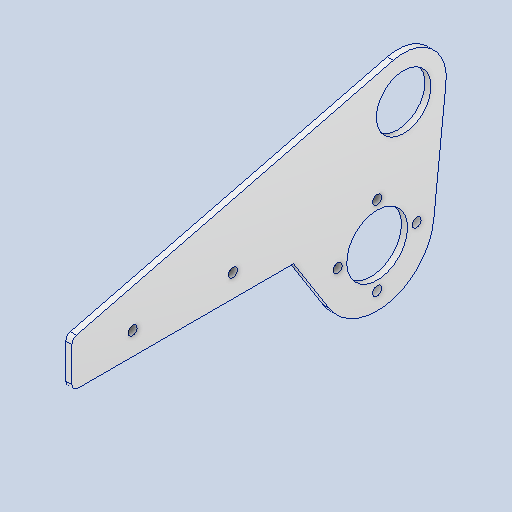
# Autodesk Inventor part: RZvector-arm-rotate-v1-Plate-MM5-F
Saved by Autodesk Inventor 2024 (Build 280153000, 153)
## iProperties
Created: 2024-03-10
Part Number: RZvector-arm-rotate-v1-Plate-MM5-F
Material: アルミニウム 6061
Document SubType Name: Modeling
Designer: haruy
Density: 2.7 g/cm^3
Appearance: アルミニウム - フラット
Mass: 7.93605 g
Surface Area: 89.4411 cm^2
Volume: 7.93605 cm^3
Author: haruy
Autodesk Inventor part; units mm, degrees
ref_plane "YZ Plane" through (0, 0, 0) normal (1, 0, 0) x (0, 1, 0)
ref_plane "XZ Plane" through (0, 0, 0) normal (0, 1, 0) x (-1, 0, 0)
ref_plane "XY Plane" through (0, 0, 0) normal (0, 0, 1) x (1, 0, 0)
derived "RZvector-arm-rotate-v1-Sketch-Base.ipt"
sketch "横から" plane through (0, 0, 0) normal (1, 0, 0) x (0, 1, 0)
  line L0 (0, 0) -> (0, -30.2937)
  line L1 (542.7807, -196.25) -> (0, -196.25)
  line L2 (628, -186.25) -> (24, -186.25)
  line L3 (24, -186.25) -> (24, -206.25)
  line L4 (24, -206.25) -> (628, -206.25)
  line L5 (628, -206.25) -> (628, -186.25)
  line L6 (138, -159.75) -> (123, -159.75)
  line L7 (123, -159.75) -> (123, -174.75)
  line L8 (123, -174.75) -> (138, -174.75)
  line L9 (138, -174.75) -> (138, -159.75)
  line L10 (0, 0) -> (0, -196.25)
  line L11 (138, -217.75) -> (123, -217.75)
  line L12 (123, -217.75) -> (123, -232.75)
  line L13 (123, -232.75) -> (138, -232.75)
  line L14 (138, -232.75) -> (138, -217.75)
  line L15 (0, 0) -> (0, -415.25)
  line L16 (54, -415.25) -> (34, -415.25)
  line L17 (34, -415.25) -> (34, -395.25)
  line L18 (34, -395.25) -> (54, -395.25)
  line L19 (54, -395.25) -> (54, -415.25)
  line L20 (134, -345.25) -> (64, -345.25)
  line L21 (64, -345.25) -> (64, -395.25)
  line L22 (64, -395.25) -> (134, -395.25)
  line L23 (134, -395.25) -> (134, -345.25)
  line L24 (136, -310.25) -> (134, -310.25)
  line L25 (134, -310.25) -> (134, -405.25)
  line L26 (134, -405.25) -> (136, -405.25)
  line L27 (136, -405.25) -> (136, -310.25)
  line L28 (136, -310.25) -> (146, -310.25)
  line L29 (146, -310.25) -> (146, -320.25)
  line L30 (146, -320.25) -> (136, -320.25)
  line L31 (136, -320.25) -> (136, -310.25)
  line L32 (146, -320.25) -> (54, -320.25)
  line L33 (54, -320.25) -> (54, -330.25)
  line L34 (54, -330.25) -> (146, -330.25)
  line L35 (146, -330.25) -> (146, -320.25)
  line L36 (0, -269) -> (385.3867, -269)
  line L37 (144, 54.75) -> (46, 54.75)
  line L38 (46, 54.75) -> (46, -139.45)
  line L39 (46, -139.45) -> (144, -139.45)
  line L40 (144, -139.45) -> (144, 54.75)
  circle A0 centre (95, 2.25) radius 95
  line L41 (176, -92.75) -> (156, -92.75)
  line L42 (156, -92.75) -> (156, -290.75)
  line L43 (156, -290.75) -> (176, -290.75)
  line L44 (176, -290.75) -> (176, -92.75)
  circle A1 centre (166, -269) radius 6
  circle A2 centre (166, -269) radius 22.5
  circle A3 centre (129.5351, -260.25) radius 15
  circle A4 centre (129.5351, -260.25) radius 6
  line L45 (138, -159.75) -> (153, -159.75)
  line L46 (153, -159.75) -> (153, -232.75)
  line L47 (153, -232.75) -> (138, -232.75)
  line L48 (138, -232.75) -> (138, -159.75)
  line L49 (123, -174.75) -> (153, -174.75)
  line L50 (153, -174.75) -> (153, -184.75)
  line L51 (153, -184.75) -> (123, -184.75)
  line L52 (123, -184.75) -> (123, -174.75)
  line L53 (123, -217.75) -> (153, -217.75)
  line L54 (153, -217.75) -> (153, -207.75)
  line L55 (153, -207.75) -> (123, -207.75)
  line L56 (123, -207.75) -> (123, -217.75)
  circle A5 centre (129.5351, -260.25) radius 18.75
  circle A6 centre (99.5351, -260.25) radius 15
  circle A7 centre (145.5, -179.75) radius 1.5
  circle A8 centre (145.5, -212.75) radius 1.5
  circle A9 centre (166, -269) radius 9
  circle A10 centre (129.5351, -260.25) radius 10
  circle A11 centre (129.5351, -260.25) radius 13
  circle A12 centre (142.5351, -260.25) radius 1.5
  circle A13 centre (129.5351, -247.25) radius 1.5
  circle A14 centre (116.5351, -260.25) radius 1.5
  circle A15 centre (129.5351, -273.25) radius 1.5
  line L57 (138, -232.75) -> (119.5367, -244.3883)
  circle A16 centre (166, -269) radius 14
  line L58 (127.5048, -278.8898) -> (164.484, -282.9177)
  line L59 (179.5784, -265.5902) -> (153, -159.75)
  line L60 (136, -330.25) -> (146, -330.25)
  line L61 (146, -330.25) -> (146, -340.25)
  line L62 (146, -340.25) -> (136, -340.25)
  line L63 (136, -340.25) -> (136, -330.25)
  line L64 (54, -405.25) -> (56, -405.25)
  line L65 (56, -405.25) -> (56, -345.2512)
  line L66 (56, -345.2512) -> (54, -345.2512)
  line L67 (54, -345.2512) -> (54, -405.25)
  line L68 (56, -320.25) -> (64.683, -320.25)
  line L69 (54, -310.25) -> (64, -310.25)
  line L70 (64, -310.25) -> (64, -320.25)
  line L71 (64, -320.25) -> (54, -320.25)
  line L72 (54, -320.25) -> (54, -310.25)
  line L73 (54, -310.25) -> (44, -310.25)
  line L74 (44, -310.25) -> (44, -340.25)
  line L75 (44, -340.25) -> (54, -340.25)
  line L76 (54, -340.25) -> (54, -310.25)
  line L77 (34, -415.25) -> (54, -415.25)
  line L78 (54, -415.25) -> (54, -139.45)
  line L79 (54, -139.45) -> (34, -139.45)
  line L80 (34, -139.45) -> (34, -415.25)
  line L81 (628, -186.25) -> (659.5, -186.25)
  line L82 (659.5, -186.25) -> (659.5, -206.25)
  line L83 (659.5, -206.25) -> (628, -206.25)
  line L84 (628, -206.25) -> (628, -186.25)
  line L85 (54, -375.25) -> (34, -375.25)
  circle A17 centre (129.5351, -260.25) radius 12.5
  circle A18 centre (643.75, -167.5) radius 15.75
  line L86 (659.5, -186.25) -> (659.5, -167.5)
  line L87 (628, -186.25) -> (628, -167.5)
  line L88 (150.5, -293.5212) -> (150.5, -446.3995)
  line L89 (34, -395.25) -> (477, -395.25)
  line L90 (477, -395.25) -> (477, -375.25)
  line L91 (477, -375.25) -> (34, -375.25)
  line L92 (34, -375.25) -> (34, -395.25)
  line L93 (184, -375.25) -> (194, -375.25)
  line L94 (194, -375.25) -> (194, -365.25)
  line L95 (194, -365.25) -> (184, -365.25)
  line L96 (184, -365.25) -> (184, -375.25)
  line L97 (230, -365.25) -> (194, -365.25)
  line L98 (194, -365.25) -> (194, -399.25)
  line L99 (194, -399.25) -> (230, -399.25)
  line L100 (230, -399.25) -> (230, -365.25)
  line L101 (212, -365.25) -> (212, -399.25)
  line L102 (194, -365.25) -> (204, -365.25)
  line L103 (204, -365.25) -> (204, -395.25)
  line L104 (204, -395.25) -> (194, -395.25)
  line L105 (194, -395.25) -> (194, -365.25)
  line L106 (423, -49.3886) -> (335, -49.3886)
  line L107 (335, -49.3886) -> (335, -349.3886)
  line L108 (335, -349.3886) -> (423, -349.3886)
  line L109 (423, -349.3886) -> (423, -49.3886)
  line L110 (394, -349.3886) -> (364, -349.3886)
  line L111 (364, -349.3886) -> (364, -369.3886)
  line L112 (364, -369.3886) -> (394, -369.3886)
  line L113 (394, -369.3886) -> (394, -349.3886)
  line L114 (359, -365.25) -> (349, -365.25)
  line L115 (349, -365.25) -> (349, -375.25)
  line L116 (349, -375.25) -> (359, -375.25)
  line L117 (359, -375.25) -> (359, -365.25)
  line L118 (379, -349.3886) -> (379, -369.3886)
  line L119 (347, -375.25) -> (357, -375.25)
  line L120 (521, -49.3886) -> (433, -49.3886)
  line L121 (433, -49.3886) -> (433, -349.3886)
  line L122 (433, -349.3886) -> (521, -349.3886)
  line L123 (521, -349.3886) -> (521, -49.3886)
  line L124 (457, -375.25) -> (447, -375.25)
  line L125 (447, -375.25) -> (447, -365.25)
  line L126 (447, -365.25) -> (457, -365.25)
  line L127 (457, -365.25) -> (457, -375.25)
  line L128 (643.186, -209.9292) -> (479.1599, -376.8167)
  line L129 (479.1599, -376.8167) -> (493.4238, -390.836)
  line L130 (493.4238, -390.836) -> (657.4499, -223.9485)
  line L131 (657.4499, -223.9485) -> (643.186, -209.9292)
  line L132 (457, -375.25) -> (457, -395.25)
  line L133 (493.1793, -362.5528) -> (507.4432, -376.5721)
  line L134 (629.1667, -224.1931) -> (643.4306, -238.2124)
  line L135 (230, -375.25) -> (220, -375.25)
  line L136 (220, -375.25) -> (220, -365.25)
  line L137 (220, -365.25) -> (230, -365.25)
  line L138 (230, -365.25) -> (230, -375.25)
  line L139 (230, -365.25) -> (65, -365.25)
  line L140 (65, -365.25) -> (65, -360.25)
  line L141 (65, -360.25) -> (230, -360.25)
  line L142 (230, -360.25) -> (230, -365.25)
  line L143 (220, -309.25) -> (65, -309.25)
  line L144 (65, -309.25) -> (65, -313.25)
  line L145 (65, -313.25) -> (220, -313.25)
  line L146 (220, -313.25) -> (220, -309.25)
  line L147 (65, -365.25) -> (70, -365.25)
  line L148 (70, -365.25) -> (70, -309.25)
  line L149 (70, -309.25) -> (65, -309.25)
  line L150 (65, -309.25) -> (65, -365.25)
  line L151 (239, -375.25) -> (239, -395.25)
  line L152 (130, -371.7504) -> (108.5351, -371.7504)
  line L153 (108.5351, -371.7504) -> (108.5351, -456.25)
  line L154 (108.5351, -456.25) -> (130, -456.25)
  line L155 (130, -456.25) -> (130, -371.7504)
  circle A19 centre (175, -269) radius 6
  line L156 (302.5611, -391.0338) -> (151.9649, -262.485)
  line L157 (151.9649, -262.485) -> (164.9496, -247.2732)
  line L158 (164.9496, -247.2732) -> (315.5458, -375.822)
  line L159 (315.5458, -375.822) -> (302.5611, -391.0338)
  circle A20 centre (427.4049, -391.1037) radius 95
  line L160 (900, 0) -> (900, -1750.1016)
  line L161 (525, -456.25) -> (0, -456.25)
  line L162 (0, -456.25) -> (0, -706.25)
  line L163 (0, -706.25) -> (525, -706.25)
  line L164 (525, -706.25) -> (525, -456.25)
  line L165 (286.9304, -332.3317) -> (437.1463, -460.5559)
  line L166 (437.1463, -460.5559) -> (497.5252, -389.8213)
  line L167 (497.5252, -389.8213) -> (347.3093, -261.5971)
  line L168 (347.3093, -261.5971) -> (286.9304, -332.3317)
  line L169 (659.5, -186.25) -> (668.5, -186.25)
  line L170 (668.5, -186.25) -> (668.5, -206.25)
  line L171 (668.5, -206.25) -> (659.5, -206.25)
  line L172 (659.5, -206.25) -> (659.5, -186.25)
  line L173 (224, -174.75) -> (194, -174.75)
  line L174 (194, -174.75) -> (194, -217.75)
  line L175 (194, -217.75) -> (224, -217.75)
  line L176 (224, -217.75) -> (224, -174.75)
  line L177 (605, -186.25) -> (605, -206.25)
  line L178 (242.3, -171.25) -> (226.4, -171.25)
  line L179 (226.4, -171.25) -> (226.4, -199.05)
  line L180 (226.4, -199.05) -> (242.3, -199.05)
  line L181 (242.3, -199.05) -> (242.3, -171.25)
  circle A21 centre (239.5, -196.25) radius 1.7
  circle A22 centre (229.2, -174.05) radius 1.7
  circle A23 centre (247.5, -196.25) radius 1.7
  line L182 (252.5, -186.25) -> (252.5, -206.25)
  line L183 (550.2984, 177.2044) -> (550.2984, -1079.3945)
  line L184 (477, -375.25) -> (590, -375.25)
  line L185 (590, -375.25) -> (590, -395.25)
  line L186 (590, -395.25) -> (477, -395.25)
  line L187 (477, -395.25) -> (477, -375.25)
  line L188 (590, -395.25) -> (578, -395.25)
  line L189 (578, -395.25) -> (578, -407.25)
  line L190 (578, -407.25) -> (590, -407.25)
  line L191 (590, -407.25) -> (590, -395.25)
  line L192 (239, -375.25) -> (229, -375.25)
  line L193 (229, -375.25) -> (229, -365.25)
  line L194 (229, -365.25) -> (239, -365.25)
  line L195 (239, -365.25) -> (239, -375.25)
  line L196 (245.8, -370.25) -> (224.6774, -352.1759)
  line L197 (224.6774, -352.1759) -> (236.9001, -337.8915)
  line L198 (236.9001, -337.8915) -> (258.0228, -355.9656)
  line L199 (258.0228, -355.9656) -> (245.8, -370.25)
  circle A24 centre (247.3784, -364.0987) radius 1.7
  circle A25 centre (237.2072, -341.8394) radius 1.7
  line L200 (239, -365.25) -> (249, -365.25)
  line L201 (249, -365.25) -> (249, -375.25)
  line L202 (249, -375.25) -> (239, -375.25)
  line L203 (239, -375.25) -> (239, -365.25)
  line L204 (249, -365.25) -> (224.6774, -365.25)
  line L205 (224.6774, -365.25) -> (224.6774, -355.25)
  line L206 (224.6774, -355.25) -> (249, -355.25)
  line L207 (249, -355.25) -> (249, -365.25)
  line L208 (224.6774, -365.25) -> (230, -365.25)
  line L209 (230, -365.25) -> (230, -375.25)
  line L210 (230, -375.25) -> (224.6774, -375.25)
  line L211 (224.6774, -375.25) -> (224.6774, -365.25)
  line L212 (224.6774, -352.1759) -> (224.6774, -355.25)
  line L213 (239, -368.75) -> (249, -368.75)
  line L214 (249, -368.75) -> (249, -371.75)
  line L215 (249, -371.75) -> (239, -371.75)
  line L216 (239, -371.75) -> (239, -368.75)
  line L217 (258.0228, -355.9656) -> (249, -375.25)
  line L218 (593.9382, -399.979) -> (576.2016, -378.5721)
  line L219 (576.2016, -378.5721) -> (590.6782, -366.5776)
  line L220 (590.6782, -366.5776) -> (608.4148, -387.9845)
  line L221 (608.4148, -387.9845) -> (593.9382, -399.979)
  circle A26 centre (596.5409, -394.1863) radius 1.7
  circle A27 centre (590.3086, -370.5201) radius 1.7
  line L222 (590, -407.25) -> (600, -407.25)
  line L223 (600, -407.25) -> (600, -397.25)
  line L224 (600, -397.25) -> (590, -397.25)
  line L225 (590, -397.25) -> (590, -407.25)
  line L226 (600, -397.25) -> (576.2016, -397.25)
  line L227 (576.2016, -397.25) -> (576.2016, -378.5721)
  line L228 (576.2016, -378.5721) -> (600, -378.5721)
  line L229 (600, -378.5721) -> (600, -397.25)
  line L230 (576.2016, -397.25) -> (578, -397.25)
  line L231 (578, -397.25) -> (578, -407.25)
  line L232 (578, -407.25) -> (576.2016, -407.25)
  line L233 (576.2016, -407.25) -> (576.2016, -397.25)
  line L234 (608.4148, -387.9845) -> (600, -407.25)
  line L235 (590, -375.25) -> (610, -375.25)
  line L236 (610, -375.25) -> (610, -395.25)
  line L237 (610, -395.25) -> (590, -395.25)
  line L238 (590, -395.25) -> (590, -375.25)
  line L239 (648.5, -186.25) -> (648.5, -206.25)
  line L240 (667.9052, -217.2444) -> (610, -371.75)
  line L241 (610, -371.75) -> (591.272, -364.7312)
  line L242 (591.272, -364.7312) -> (649.1773, -210.2256)
  line L243 (649.1773, -210.2256) -> (667.9052, -217.2444)
  line L244 (660.8864, -235.9723) -> (642.1585, -228.9535)
  line L245 (617.0188, -353.022) -> (598.2909, -346.0032)
  point P0 (166, -92.75)
  point P1 (176, -259.202)
  point P2 (176, -251.3403)
  point P3 (394, -359.3886)
  point P4 (643.75, -206.25)
  point P5 (247.4615, -346.9286)
  dimension "d9" = 26
  dimension "d1" = 3
  dimension "d2" = 3
  dimension "d3" = 7.5
  dimension "d4" = 7.5
  dimension "d5" = 5
  dimension "d6" = 5
  dimension "d7" = 18
  dimension "d8" = 20
  dimension "d10" = 3
  dimension "d13" = 360
  dimension "d17" = 28
  measures "d1" diameter of A7
  measures "d2" diameter of A8
  measures "d3" distance from line of A7.centre L48
  measures "d4" distance from line of A8.centre L48
  measures "d5" distance from line of A8.centre L55
  measures "d6" distance from line of A7.centre L51
  measures "d7" diameter of A9
  measures "d8" diameter of A10
  measures "d10" diameter of A12
  measures "d17" diameter of A16
extrude "押し出し1" add sketch "横から" along normal blind 2 contours L158 L44 L59 | L59 A19 A16 L44 L158 | L59 A2 L42 L4 | L4 L42 L1 L59 | A16 A19 L44 L36 | L36 L44 A19 A16 | L59 A16 A19 | A16 L44 A19 | L44 L158 L157 L42 A2 L59 | L44 A16 L42 L157 L158 | L42 A2 A5 L57 L47 L46 L4 | L4 L46 L1 L42 | L1 L42 L2 L59 | L44 A19 A9 L36 | L36 A9 A19 L44 | A19 L44 A16 | A16 L156 A9 A19 L44 | A16 L42 L36 A9 L156 | L42 L157 L156 A16 L36 A5 A2 | L44 A19 A9 L156 L42 A16 | L2 L42 L59 | L46 L55 L48 L4 | L4 L48 L1 L46 | L1 L46 L2 L42 | L58 L42 A16 | L42 A16 L156 L157 | A5 L36 A2 | A2 A3 A6 A5 | L42 L156 A16 | L2 L46 L59 L42 | L1 L48 L2 L46 | L46 L53 L48 L55 | A16 L36 L42 | L42 L58 A2 A5 L36 A16 | L36 L42 L156 A9 | A2 L36 A3 | A3 L36 A11 A12 A13 A14 | L42 L36 A16 L156 | L2 L48 L51 L46 | L46 L49 L9 L45 | L46 L47 L14 L53 | L58 A5 A2 | A2 A5 L36 A3 | L36 A5 A2 | A3 L36 A11 A15 | A6 A5 | L51 L48 L49 L46 | A11 A15 A17 L36 | L36 A17 A12 A11 | L36 A5 A6 A3 | A17 A15 L36 A10 | L36 A10 A17 A14 A13 A12 | A11 A14 A17 L36 | L36 A17 A15 A11 | A17 A13 A11 A12 | A11 A13 A17 A14
fillet "フィレット1" radius 2 2 edges at (1, 153, -159.75) (1, 138, -159.75)
equation "\"d4\" = d3"
